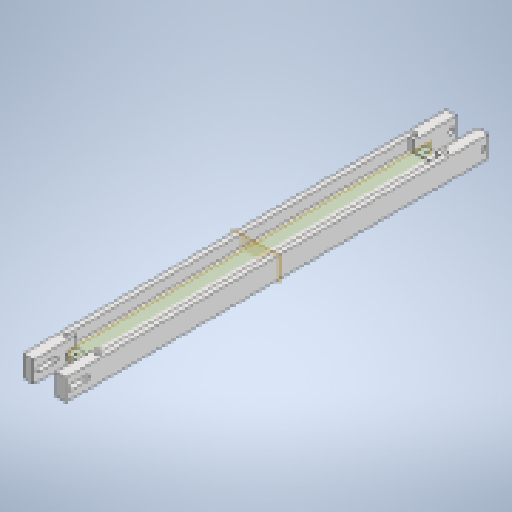
# Autodesk Inventor part: Sledge_rail
Saved by Autodesk Inventor 2025.1 (Build 291241020, 241B)
## iProperties
Created: 2024-11-07
Part Number: Sledge_rail
Material: Generic
Document SubType Name: Modeling
Designer: leon-
Density: 1 g/cm^3
Appearance: Default
Author: leon-
Autodesk Inventor part; units mm, degrees
ref_plane "YZ Plane" through (0, 0, 0) normal (1, 0, 0) x (0, 1, 0)
ref_plane "XZ Plane" through (0, 0, 0) normal (0, 1, 0) x (-1, 0, 0)
ref_plane "XY Plane" through (0, 0, 0) normal (0, 0, 1) x (1, 0, 0)
sketch "Sketch1" plane through (0, 0, 0) normal (0, 0, 1) x (1, 0, 0)
  line L0 (0, 0) -> (20, 0)
  line L1 (20, 0) -> (20, 16)
  line L2 (20, 16) -> (15, 16)
  line L3 (15, 16) -> (15, 5)
  line L4 (15, 5) -> (0, 5)
  line L5 (0, 5) -> (0, 0)
  line L6 (20, 0) -> (15, 0)
  line L7 (15, 0) -> (15, -4)
  line L8 (15, -4) -> (20, -4)
  line L9 (20, -4) -> (20, 0)
  dimension "d0" = 5
  dimension "d1" = 20
  dimension "d2" = 5
  dimension "d3" = 16
  dimension "d4" = 20
  constraints: 20 end point, 6 perpendicular, 2 horizontal, 2 parallel, 1 collinear
  measures "d0" distance between parallel lines of L1 L3
  measures "d1" distance between parallel lines of L5 L1
  measures "d2" distance between parallel lines of L0 L4
  measures "d3" distance between parallel lines of L0 L2
  measures "d4" distance from line of L8 L2.end
extrude "Extrusion1" add sketch "Sketch1" along normal blind 320
mirror "Mirror1" about plane through (0, 0, 0) normal (1, 0, 0) of "Extrusion1"
ref_plane "Work Plane1" through (0, 0, 160) normal (0, 0, 1) x (1, 0, 0)
sketch "Sketch3" plane through (0, 0, 0) normal (0, 0, -1) x (-1, 0, 0)
  line L0 (20, -4) -> (20, 16) projected
  line L1 (-15, -4) -> (-20, -4) projected
  line L2 (20, 16) -> (-20, 16)
  line L3 (-20, 16) -> (-20, -4)
  line L4 (-20, -4) -> (20, -4)
  line L5 (20, -4) -> (20, 16)
  point P0 (0, 0)
  constraints: 8 end point, 2 parallel, 1 horizontal, 1 perpendicular
extrude "Extrusion2" add sketch "Sketch3" along normal blind 10
ref_plane "Work Plane2" through (0, -4, 320) normal (-1, 0, 0) x (0, 0, 1)
sketch "Sketch4" plane through (-15, 16, 0) normal (0, 1, 0) x (1, 0, 0)
  line L0 (15, -386) -> (15, 76) projected
  point P0 (15, 0)
  point P1 (0, 4.6383)
  point P2 (30, 4.6383)
  dimension "d9" = 30
  dimension "d10" = 15
  measures "d9" distance of point (30, 4.638) point (0, 4.638)
  measures "d10" distance from line of L0 point (30, 4.638)
hole "Hole1" at (-15, 16, -4.6383) at (15, 16, -4.6383) direction (0, -1, 0) diameter 5 end through all
mirror "Mirror3" about plane through (0, 0, 160) normal (0, 0, 1) of "Extrusion2", "Hole1"
sketch "Sketch5" plane through (-20, 16, -10) normal (0, 1, 0) x (1, 0, 0)
  line L0 (35, -330) -> (5, -330) projected
  line L1 (0, -340) -> (40, -340) projected
  line L2 (30, -330) -> (10, -330)
  line L3 (10, -330) -> (10, -340)
  line L4 (10, -340) -> (30, -340)
  line L5 (30, -340) -> (30, -330)
  line L6 (20, -396) -> (20, 66) projected
  point P0 (20, -10)
  point P1 (20, -340)
  point P2 (20, -330)
  dimension "d18" = 20
  dimension "d31" = 10
  constraints: 8 end point, 2 parallel, 2 point on line, 1 horizontal, 1 perpendicular
  measures "d18" distance between parallel lines of L3 L5
  measures "d31" distance between parallel lines of L6 L5
extrude "Extrusion3" cut sketch "Sketch5" against normal blind 10
sketch "Sketch6" plane through (-20, 6, -10) normal (0, 1, 0) x (1, 0, 0)
  line L0 (30, -340) -> (10, -340) projected
  line L1 (30, -330) -> (30, -340) projected
  point P0 (20, -10)
  point P1 (24.8, -336)
  point P2 (15.3, -336)
  dimension "d21" = 4
  dimension "d22" = 9.5
  dimension "d30" = 5.2
  constraints: 1 horizontal alignment
  measures "d21" distance from line of L0 point (24.8, -336)
  measures "d22" distance of point (15.3, -336) point (24.8, -336)
  measures "d30" distance from line of point (24.8, -336) L1
hole "Hole2" at (4.8, 6, 326) at (-4.7, 6, 326) direction (0, -1, 0) diameter 2.3 end through all
mirror "Mirror4" about plane through (0, 0, 160) normal (0, 0, 1) of "Hole2", "Extrusion3"
sketch "Sketch7" plane through (-20, -4, 330) normal (0, 0, 1) x (1, 0, 0)
  line L0 (10, 20) -> (10, 10) projected
  line L1 (10, 20) -> (0, 20)
  line L2 (0, 20) -> (0, 0)
  line L3 (0, 0) -> (10, 0)
  line L4 (10, 0) -> (10, 20)
  line L5 (40, 0) -> (0, 0) projected
  line L6 (0, 0) -> (0, 20) projected
  point P0 (20, 4)
  point P1 (10, 10)
  constraints: 8 end point, 2 collinear, 2 parallel, 1 horizontal, 1 perpendicular
extrude "Extrusion4" add sketch "Sketch7" along normal blind 30
mirror "Mirror6" about plane through (0, 0, 160) normal (0, 0, 1) of "Extrusion4"
mirror "Mirror7" about plane through (0, -4, 320) normal (-1, 0, 0) of "Extrusion4", "Mirror6"
sketch "Sketch10" plane through (-10, -4, 330) normal (1, 0, 0) x (0, 0, -1)
  line L0 (-10, 10) -> (-25, 10) construction
  line L1 (-10, 12.5) -> (-25, 12.5)
  line L2 (-25, 7.5) -> (-10, 7.5)
  arc A0 (-10, 7.5) -> (-10, 12.5) centre (-10, 10) ccw
  arc A1 (-25, 12.5) -> (-25, 7.5) centre (-25, 10) ccw
  line L3 (-30, 0) -> (-30, 20) projected
  line L4 (0, 0) -> (-30, 0) projected
  point P0 (330, 4)
  point P1 (-17.5, 10)
  dimension "d45" = 2.5
  dimension "d46" = 15
  dimension "d47" = 5
  dimension "d48" = 10
  constraints: 8 end point, 4 point on circle, 4 tangent, 2 centre point, 1 horizontal, 1 midpoint, 1 parallel
  measures "d45" radius of A1
  measures "d46" distance of L2.start L2.end
  measures "d47" distance from line of L3 L0.end
  measures "d48" distance between parallel lines of L4 L0
extrude "Extrusion6" cut sketch "Sketch10" against normal through all
mirror "Mirror5" about plane through (0, -4, 320) normal (-1, 0, 0) of "Extrusion4", "Extrusion6"
sketch "Sketch9" plane through (-20, -4, -10) normal (0, -1, 0) x (1, 0, 0)
  line L0 (10, 340) -> (10, 370) projected
  line L1 (30, 330) -> (30, 340) projected
  line L2 (10, 340) -> (30, 340)
  line L3 (30, 340) -> (30, 330)
  line L4 (30, 330) -> (10, 330)
  line L5 (10, 330) -> (10, 340)
  point P0 (20, 10)
  constraints: 8 end point, 2 parallel, 1 horizontal, 1 perpendicular
extrude "Extrusion5" cut sketch "Sketch9" against normal up to surface (4 mm away)
sketch "Sketch11" plane through (-20, -4, 360) normal (-1, 0, 0) x (0, 0, 1)
  line L0 (-400, 20) -> (-400, 0) projected
  line L1 (0, 20) -> (-400, 20) projected
  point P0 (-360, 4)
  point P1 (-395, 10)
  point P2 (-400, 10)
  dimension "d51" = 5
  dimension "d52" = 10
  constraints: 1 midpoint
  measures "d51" distance of point (-400, 10) point (-395, 10)
  measures "d52" distance from line of L1 point (-395, 10)
hole "Hole4" at (-20, 6, -35) direction (1, 0, 0) diameter 5 end through all
equation "\"d10\" = 0.5 * d9"
body "Solid1"
